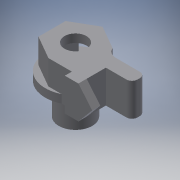
# Autodesk Inventor part: wingnut_final
Saved by Autodesk Inventor 2018 (Build 220112000, 112)
## iProperties
Created: 2017-11-02
Part Number: wingnut_final
Material: Generic
Document SubType Name: Modeling
Designer: Payal Jindal
Density: 1 g/cm^3
Appearance: Default
Author: Payal Jindal
Autodesk Inventor part; units mm, degrees
ref_plane "YZ Plane" through (0, 0, 0) normal (1, 0, 0) x (0, 1, 0)
ref_plane "XZ Plane" through (0, 0, 0) normal (0, 1, 0) x (-1, 0, 0)
ref_plane "XY Plane" through (0, 0, 0) normal (0, 0, 1) x (1, 0, 0)
sketch "Sketch1" plane through (0, 0, 0) normal (0, 0, 1) x (1, 0, 0)
  line L0 (0, 6.4158) -> (5.5563, 3.2079)
  line L1 (5.5563, 3.2079) -> (5.5562, -3.2079)
  line L2 (5.5562, -3.2079) -> (0, -6.4158)
  line L3 (0, -6.4158) -> (-5.5562, -3.2079)
  line L4 (-5.5562, -3.2079) -> (-5.5563, 3.2079)
  line L5 (-5.5563, 3.2079) -> (0, 6.4158)
  line L6 (8.5562, 4.94) -> (0, 9.8799)
  line L7 (0, 9.8799) -> (-8.5563, 4.94)
  line L8 (-8.5563, 4.94) -> (-8.5562, -4.94)
  line L9 (-8.5562, -4.94) -> (0, -9.8799)
  line L10 (0, -9.8799) -> (8.5563, -4.94)
  line L11 (8.5563, -4.94) -> (8.5562, 4.94)
  line L12 (5.5563, 3.2079) -> (5.5563, 6.672)
  line L13 (8.5562, 4.94) -> (5.5563, 6.672)
  line L14 (-5.5563, 3.2079) -> (-5.5563, 6.672)
  line L15 (-8.5563, 4.94) -> (-5.5563, 6.672)
  point P0 (0, 0)
  point P1 (0, 0)
  dimension "d0" = 5.5563
  dimension "d1" = 3
  constraints: 32 end point, 2 point on line, 2 vertical, 1 coincident, 1 collinear, 1 parallel, 18 other
  measures "d0" distance from line of L0 point (0, 0)
  measures "d1" distance between parallel lines of L0 L6
sketch "Sketch2" plane through (0, 0, 0) normal (0, 0, 1) x (1, 0, 0)
  line L0 (8.5562, 4.94) -> (0, 9.8799) projected
  line L1 (0, 9.8799) -> (-8.5563, 4.94) projected
  line L2 (-8.5563, 4.94) -> (-8.5562, -4.94) projected
  line L3 (-8.5562, -4.94) -> (0, -9.8799) projected
  line L4 (0, -9.8799) -> (8.5563, -4.94) projected
  line L5 (8.5563, -4.94) -> (8.5562, 4.94) projected
  point P0 (0, 0)
extrude "Extrusion1" add sketch "Sketch2" against normal blind 3
extrude "Extrusion2" add sketch "Sketch1" along normal blind 2.9766 contours L12 L6 L11 L10 L9 L8 L7 L14 L4 L3 L2 L1
mirror "Mirror1" about plane through (0, -1.6917, 2.9766) normal (0, 0, 1) of "Extrusion2", "Extrusion1"
sketch "Sketch3" plane through (-8.5562, -4.94, 8.9531) normal (0, 0, 1) x (1, 0, 0)
  line L0 (8.5562, 14.8199) -> (17.1125, 9.8799) projected
  line L1 (0, 9.8799) -> (8.5562, 14.8199) projected
  line L2 (0, 0) -> (0, 9.8799) projected
  line L3 (8.5562, -4.94) -> (0, 0) projected
  line L4 (17.1125, 0) -> (8.5562, -4.94) projected
  line L5 (17.1125, 9.8799) -> (17.1125, 0) projected
  point P0 (8.5563, 4.94)
hole "Hole1" at (0, 0, 8.9531) direction (0, 0, -1) diameter 8 end up to face face through (2.8521, -1.6467, -3) facing (0, 0, -1)
sketch "Sketch5" plane through (0, 0, -3) normal (0, 0, -1) x (-1, 0, 0)
  line L0 (-8.5562, 4.94) -> (-8.5563, -4.94) projected
  line L1 (-8.5563, -2.45) -> (-8.5563, 2.45)
  line L2 (-8.5563, 2.45) -> (-23, 2.45)
  line L3 (-23, 2.45) -> (-23, -2.45)
  line L4 (-23, -2.45) -> (-8.5563, -2.45)
  point P0 (0, 0)
  point P1 (-8.5563, 0)
  dimension "d16" = 23
  dimension "d17" = 4.9
  constraints: 8 end point, 2 midpoint, 2 parallel, 2 point on line, 1 perpendicular
  measures "d16" distance from line of point (0, 0) L3
  measures "d17" distance of L2.end L3.end
extrude "Extrusion4" add sketch "Sketch5" against normal up to surface (11.9531 mm away)
sketch "Sketch6" plane through (8.5563, -2.45, -3) normal (0, -1, 0) x (1, 0, 0)
  line L0 (0, 11.9531) -> (-8.5562, 11.9531) projected
  line L1 (0, 0) -> (0, 11.9531) projected
  line L2 (0, 11.9531) -> (0, 0)
  line L3 (0, 0) -> (4.9437, 0)
  line L4 (4.9437, 0) -> (4.9437, 11.9531)
  line L5 (4.9437, 11.9531) -> (0, 11.9531)
  line L6 (14.4437, 0) -> (14.4437, 11.9531) projected
  point P0 (-8.5563, 3)
  dimension "d20" = 9.5
  constraints: 8 end point, 2 parallel, 1 perpendicular, 1 vertical
  measures "d20" distance between parallel lines of L4 L6
extrude "Extrusion5" add sketch "Sketch6" along normal blind 10
sketch "Sketch9" plane through (8.5563, -12.45, -3) normal (0, -1, 0) x (1, 0, 0)
  line L0 (4.9437, 11.9531) -> (4.9437, 0) projected
  line L1 (4.9437, 5.9766) -> (9.9437, 5.9766) construction
  line L2 (9.9437, 5.9766) -> (4.9437, 0)
  line L3 (9.9437, 5.9766) -> (4.9437, 11.9531)
  point P0 (-8.5563, 3)
  dimension "d24" = 5
  constraints: 6 end point, 1 horizontal, 1 midpoint
  measures "d24" distance of L1.start L1.end
extrude "Extrusion6" add sketch "Sketch9" against normal blind 3
sketch "Sketch10" plane through (8.5563, -12.45, -3) normal (-1, 0, 0) x (0, 0, 1)
  line L0 (0, 2.5701) -> (11.9531, 2.5701) projected
  line L1 (11.9531, 7.51) -> (11.9531, 0) projected
  line L2 (0, 7.51) -> (11.9531, 7.51) projected
  line L3 (0, 7.51) -> (0, 0) projected
  point P0 (3, 12.45)
extrude "Extrusion7" add sketch "Sketch10" along normal up to surface surface through (8.5563, -4.94, 0) normal (0.5, -0.8660254, 0)
fillet "Fillet1" radius 4 1 edges at (8.5563, 2.45, 2.9766)
fillet "Fillet2" radius 2 2 edges at (23, -2.45, 2.9766) (23, 2.45, 2.9766)
sketch "Sketch11" plane through (0, 0, -3) normal (0, 0, -1) x (-1, 0, 0)
  circle A0 centre (0, 0) radius 6.096
  circle A1 centre (0, 0) radius 4 projected
  circle A2 centre (0, 0) radius 4
  dimension "d31" = 12.192
  constraints: 2 centre point, 2 coincident, 1 concentric
  measures "d31" diameter of A0
extrude "Extrusion8" add sketch "Sketch11" along normal blind 11.3538
sketch "Sketch12" plane through (0, 0, -3) normal (0, 0, -1) x (-1, 0, 0)
  circle A0 centre (0, 0) radius 11
  dimension "d34" = 22
  constraints: 1 centre point, 1 coincident
  measures "d34" diameter of A0
extrude "Extrusion9" add sketch "Sketch12" against normal up to surface (3 mm away)
body "Solid1"
